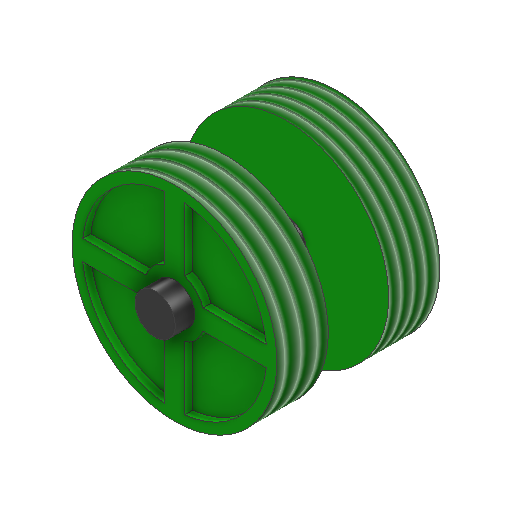
# Autodesk Inventor part: Coletor - Hand
Saved by Autodesk Inventor 2025.3 (Build 293356000, 356)
## iProperties
Created: 2026-05-13
Part Number: Coletor - Hand
Material: Genérico
Document SubType Name: Modeling
Designer: djair.oliveira
Density: 1 g/cm^3
Appearance: Padrão
Author: djair.oliveira
Autodesk Inventor part; units mm, degrees
ref_plane "YZ Plane" through (0, 0, 0) normal (1, 0, 0) x (0, 1, 0)
ref_plane "XZ Plane" through (0, 0, 0) normal (0, 1, 0) x (-1, 0, 0)
ref_plane "XY Plane" through (0, 0, 0) normal (0, 0, 1) x (1, 0, 0)
sketch "Esboço1" plane through (0, 0, 0) normal (1, 0, 0) x (0, 1, 0)
  line L0 (0, 0) -> (0, 100)
  line L1 (0, 100) -> (10, 100)
  line L2 (10, 100) -> (10, 90.4)
  line L3 (10, 90.4) -> (50.8, 90.4)
  line L4 (50.8, 90.4) -> (50.8, 65)
  line L5 (50.8, 65) -> (10, 65)
  line L6 (10, 65) -> (10, 35)
  line L7 (10, 35) -> (50.8, 35)
  line L8 (50.8, 35) -> (50.8, 9.6)
  line L9 (50.8, 9.6) -> (10, 9.6)
  line L10 (10, 9.6) -> (10, 0)
  line L11 (10, 0) -> (0, 0)
  line L12 (0, 50) -> (10, 50)
  dimension "d0" = 10
  dimension "d1" = 100
  dimension "d2" = 25.4
  dimension "d3" = 25.4
  dimension "d4" = 15
  dimension "d5" = 15
  dimension "d6" = 50.8
  constraints: 26 end point, 8 perpendicular, 6 point on line, 2 midpoint, 1 horizontal, 1 vertical
  measures "d0" distance of L10.end L0.start
  measures "d1" distance of L0.start L0.end
  measures "d2" distance of L3.end L4.end
  measures "d3" distance of L7.end L8.end
  measures "d4" distance between parallel lines of L5 L12
  measures "d5" distance between parallel lines of L12 L7
  measures "d6" distance between parallel lines of L0 L4
revolve "Revolução1" add sketch "Esboço1" angle 360 about axis through (0, 0, 0) along (0, 0, 1)
thread "Rosca1" size "M1060x8" class "6g" standard "ANSI Metric M Profile" full length
thread "Rosca2" size "M105x6" class "6g" standard "ANSI Metric M Profile" full length
sketch "Esboço2" plane through (0, 0, 90.4) normal (0, 0, 1) x (1, 0, 0)
  circle A0 centre (0, 0) radius 10 projected
  circle A1 centre (0, 0) radius 45.8
  circle A2 centre (0, 0) radius 50.8 projected
  circle A3 centre (0, 0) radius 15
  line L0 (50.5533, 5) -> (-50.5533, 5)
  line L1 (-50.5533, 5) -> (-50.5533, -5)
  line L2 (-50.5533, -5) -> (50.5533, -5)
  line L3 (50.5533, -5) -> (50.5533, 5)
  line L4 (50.5533, 5) -> (-50.5533, -5) construction
  line L5 (-50.5533, 5) -> (50.5533, -5) construction
  line L6 (5, 50.5533) -> (-5, 50.5533)
  line L7 (-5, 50.5533) -> (-5, -50.5533)
  line L8 (-5, -50.5533) -> (5, -50.5533)
  line L9 (5, -50.5533) -> (5, 50.5533)
  line L10 (5, 50.5533) -> (-5, -50.5533) construction
  line L11 (-5, 50.5533) -> (5, -50.5533) construction
  point P0 (5, 45.5263)
  point P1 (5, 14.1421)
  point P2 (14.1421, 5)
  point P3 (45.5263, 5)
  point P4 (5, -14.1421)
  point P5 (5, -45.5263)
  point P6 (45.5263, -5)
  point P7 (14.1421, -5)
  point P8 (-5, 14.1421)
  point P9 (-5, 45.5263)
  point P10 (-45.5263, 5)
  point P11 (-14.1421, 5)
  point P12 (-5, -45.5263)
  point P13 (-5, -14.1421)
  point P14 (-14.1421, -5)
  point P15 (-45.5263, -5)
  dimension "d12" = 5
  dimension "d13" = 5
  dimension "d14" = 10
  dimension "d15" = 10
  constraints: 24 end point, 4 midpoint, 4 parallel, 2 centre point, 2 coincident, 2 horizontal, 2 perpendicular, 2 point on circle
  measures "d12" radial gap between concentric circles of A2 A1
  measures "d13" radial gap between concentric circles of A3 A0
  measures "d14" distance between parallel lines of L2 L0
  measures "d15" distance between parallel lines of L7 L9
extrude "Extrusão1" cut sketch "Esboço2" against normal blind 4 contours A3 L9 A1 L0 | L2 A1 L9 A3 | A3 L0 A1 L7 | L7 A1 L2 A3
sketch "Esboço3" plane through (0, 0, 9.6) normal (0, 0, -1) x (-1, 0, 0)
  circle A0 centre (0, 0) radius 10 projected
  arc A1 (45.5263, 5) -> (5, 45.5263) centre (0, 0) ccw projected
  line L0 (14.1421, 5) -> (45.5263, 5) projected
  arc A2 (14.1421, 5) -> (5, 14.1421) centre (0, 0) ccw projected
  line L1 (5, 45.5263) -> (5, 14.1421) projected
  arc A3 (5, -14.1421) -> (14.1421, -5) centre (0, 0) ccw projected
  line L2 (45.5263, -5) -> (14.1421, -5) projected
  arc A4 (5, -45.5263) -> (45.5263, -5) centre (0, 0) ccw projected
  line L3 (5, -14.1421) -> (5, -45.5263) projected
  arc A5 (-45.5263, -5) -> (-5, -45.5263) centre (0, 0) ccw projected
  line L4 (-14.1421, -5) -> (-45.5263, -5) projected
  arc A6 (-14.1421, -5) -> (-5, -14.1421) centre (0, 0) ccw projected
  line L5 (-5, -45.5263) -> (-5, -14.1421) projected
  arc A7 (-5, 14.1421) -> (-14.1421, 5) centre (0, 0) ccw projected
  line L6 (-45.5263, 5) -> (-14.1421, 5) projected
  arc A8 (-5, 45.5263) -> (-45.5263, 5) centre (0, 0) ccw projected
  line L7 (-5, 14.1421) -> (-5, 45.5263) projected
extrude "Extrusão2" cut sketch "Esboço3" against normal blind 4 contours L0 A2 L1 A1 | A3 L2 A4 L3 | L4 A6 L5 A5 | A7 L6 A8 L7
equation "\"d3\" = d2"
equation "\"d5\" = d4"
equation "\"d15\" = d14"
